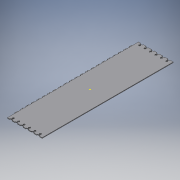
# Autodesk Inventor part: 3DPrinterBracket_bottom
Saved by Autodesk Inventor 2016 (Build 200138000, 138)
## iProperties
Created: 2017-10-03
Part Number: 3DPrinterBracket_bottom
Material: Generic
Document SubType Name: Modeling
Designer: jcj2131
Density: 1 g/cm^3
Appearance: Default
Author: jcj2131
Autodesk Inventor part; units mm, degrees
ref_plane "YZ Plane" through (0, 0, 0) normal (1, 0, 0) x (0, 1, 0)
ref_plane "XZ Plane" through (0, 0, 0) normal (0, 1, 0) x (-1, 0, 0)
ref_plane "XY Plane" through (0, 0, 0) normal (0, 0, 1) x (1, 0, 0)
sketch "Sketch1" plane through (0, 0, 0) normal (0, 1, 0) x (-1, 0, 0)
  line L0 (82.55, 306.3875) -> (-82.55, 306.3875)
  line L1 (-82.55, 306.3875) -> (-82.55, -306.3875)
  line L2 (-82.55, -306.3875) -> (82.55, -306.3875)
  line L3 (82.55, -306.3875) -> (82.55, 306.3875)
  point P0 (0, 0)
  point P1 (0, 306.3875)
  point P2 (82.55, 0)
  dimension "d0" = 612.775
  dimension "d1" = 165.1
  constraints: 8 end point, 2 midpoint, 2 parallel, 1 horizontal, 1 horizontal alignment, 1 perpendicular, 1 vertical alignment
  measures "d0" distance of L2.end L0.start
  measures "d1" distance of L0.start L0.end
extrude "Extrusion1" add sketch "Sketch1" along normal blind 3.175
sketch "Sketch2" plane through (0, 3.175, 0) normal (0, 1, 0) x (1, 0, 0)
  line L0 (-82.55, -306.3875) -> (82.55, -306.3875) projected
  line L1 (-69.85, -306.3875) -> (-57.15, -306.3875)
  line L2 (-57.15, -306.3875) -> (-57.15, -303.2125)
  line L3 (-57.15, -303.2125) -> (-69.85, -303.2125)
  line L4 (-69.85, -303.2125) -> (-69.85, -306.3875)
  line L5 (-82.55, 306.3875) -> (-82.55, -306.3875) projected
  point P0 (0, 0)
  dimension "d4" = 12.7
  dimension "d5" = 12.7
  dimension "d6" = 3.175
  constraints: 8 end point, 2 parallel, 1 horizontal, 1 perpendicular, 1 point on line
  measures "d4" distance between parallel lines of L5 L4
  measures "d5" distance of L2.end L3.end
  measures "d6" distance of L1.end L2.end
extrude "Extrusion2" cut sketch "Sketch2" against normal through all
sketch "Sketch3" plane through (0, 3.175, 0) normal (0, 1, 0) x (1, 0, 0)
  line L0 (-57.15, -303.2125) -> (-69.85, -303.2125) projected
  line L1 (-65.278, -303.2125) -> (-61.722, -303.2125)
  line L2 (-61.722, -303.2125) -> (-61.722, -297.2125)
  line L3 (-61.722, -297.2125) -> (-65.278, -297.2125)
  line L4 (-65.278, -297.2125) -> (-65.278, -303.2125)
  line L5 (-69.85, -306.3875) -> (-69.85, -303.2125) projected
  point P0 (0, 0)
  dimension "d9" = 3.556
  dimension "d10" = 6
  dimension "d11" = 4.572
  constraints: 8 end point, 2 parallel, 1 horizontal, 1 perpendicular, 1 point on line
  measures "d9" distance of L2.end L3.end
  measures "d10" distance of L3.end L1.start
  measures "d11" distance between parallel lines of L5 L4
extrude "Extrusion3" cut sketch "Sketch3" against normal through all
sketch "Sketch4" plane through (0, 3.175, 0) normal (0, 1, 0) x (1, 0, 0)
  line L0 (-59.5315, -297.2125) -> (-67.469, -297.2125)
  line L1 (-67.469, -297.2125) -> (-67.469, -294.4345)
  line L2 (-67.469, -294.4345) -> (-59.5315, -294.4345)
  line L3 (-59.5315, -294.4345) -> (-59.5315, -297.2125)
  line L4 (-65.278, -297.2125) -> (-61.722, -297.2125) projected
  line L5 (-69.85, -306.3875) -> (-69.85, -303.2125) projected
  point P0 (0, 0)
  dimension "d14" = 7.9375
  dimension "d15" = 2.778
  dimension "d16" = 0
  dimension "d17" = 2.381
  constraints: 8 end point, 2 parallel, 1 horizontal, 1 perpendicular
  measures "d14" distance of L1.end L2.end
  measures "d15" distance of L0.end L1.end
  measures "d16" distance between parallel lines of L4 L0
  measures "d17" distance between parallel lines of L5 L1
extrude "Extrusion4" cut sketch "Sketch4" against normal through all
sketch "Sketch5" plane through (0, 3.175, 0) normal (0, 1, 0) x (1, 0, 0)
  line L0 (-59.5315, -294.4345) -> (-67.469, -294.4345) projected
  line L1 (-65.278, -294.4345) -> (-61.722, -294.4345)
  line L2 (-61.722, -294.4345) -> (-61.722, -291.1475)
  line L3 (-61.722, -291.1475) -> (-65.278, -291.1475)
  line L4 (-65.278, -291.1475) -> (-65.278, -294.4345)
  line L5 (-69.85, -306.3875) -> (-69.85, -303.2125) projected
  line L6 (-57.15, -306.3875) -> (82.55, -306.3875) projected
  point P0 (0, 0)
  dimension "d20" = 3.556
  dimension "d21" = 4.572
  dimension "d22" = 15.24
  constraints: 8 end point, 2 parallel, 1 horizontal, 1 perpendicular, 1 point on line
  measures "d20" distance of L2.end L3.end
  measures "d21" distance between parallel lines of L5 L4
  measures "d22" distance between parallel lines of L6 L3
extrude "Extrusion5" cut sketch "Sketch5" against normal through all
pattern_linear "Rectangular Pattern1" count 6 spacing 25.4 along (1, 0, 0) of "Extrusion2", "Extrusion3", "Extrusion4", "Extrusion5"
sketch "Sketch6" plane through (0, 3.175, 0) normal (0, 1, 0) x (1, 0, 0)
  point P0 (0, 0)
mirror "Mirror1" about plane through (0, 0, 0) normal (0, 0, 1) of "Extrusion5", "Extrusion2", "Extrusion3", "Extrusion4", "Rectangular Pattern1"
sketch "Sketch18" plane through (0, 3.175, 0) normal (0, 1, 0) x (1, 0, 0)
  line L0 (-46.25, 241.3875) -> (-6.25, 241.3875)
  line L1 (-6.25, 241.3875) -> (-6.25, 281.3875)
  line L2 (-6.25, 281.3875) -> (-46.25, 281.3875)
  line L3 (-46.25, 281.3875) -> (-46.25, 241.3875)
  line L4 (82.55, -306.3875) -> (82.55, 306.3875) projected
  line L5 (-19.05, 306.3875) -> (-31.75, 306.3875) projected
  point P0 (0, 0)
  dimension "d120" = 40
  dimension "d121" = 40
  dimension "d122" = 128.8
  dimension "d123" = 25
  constraints: 8 end point, 2 parallel, 1 horizontal, 1 perpendicular
  measures "d120" distance of L2.end L0.start
  measures "d121" distance of L1.end L2.end
  measures "d122" distance between parallel lines of L4 L3
  measures "d123" distance between parallel lines of L5 L2
extrude "Extrusion13" [suppressed]
sketch "Sketch19" plane through (0, 3.175, 0) normal (0, 1, 0) x (1, 0, 0)
  circle A0 centre (-60.6, 251.3875) radius 2.75
  line L0 (-6.25, 241.3875) -> (-46.25, 241.3875) projected
  circle A1 centre (-60.6, 271.3875) radius 2.75
  line L1 (-46.25, 281.3875) -> (-46.25, 241.3875) projected
  point P0 (0, 0)
  dimension "d126" = 5.5
  dimension "d127" = 10
  dimension "d128" = 5.5
  dimension "d129" = 20
  dimension "d130" = 14.35
  dimension "d131" = 14.35
  constraints: 2 centre point
  measures "d126" diameter of A0
  measures "d127" distance from line of L0 A0.centre
  measures "d128" diameter of A1
  measures "d129" distance of A0.centre A1.centre
  measures "d130" distance from line of L1 A0.centre
  measures "d131" distance from line of L1 A1.centre
extrude "Extrusion14" [suppressed]
sketch "Sketch20" plane through (0, 3.175, 0) normal (0, 1, 0) x (1, 0, 0)
  line L0 (-82.55, -306.3875) -> (-69.85, -306.3875) projected
  line L1 (-82.55, -306.3875) -> (-79.375, -306.3875)
  line L2 (-79.375, -306.3875) -> (-79.375, -268.2875)
  line L3 (-79.375, -268.2875) -> (-82.55, -268.2875)
  line L4 (-82.55, -268.2875) -> (-82.55, -306.3875)
  line L5 (-82.55, 306.3875) -> (-82.55, -306.3875) projected
  line L6 (-82.55, -263.7155) -> (-79.375, -263.7155)
  line L7 (-79.375, -263.7155) -> (-79.375, -260.1595)
  line L8 (-79.375, -260.1595) -> (-82.55, -260.1595)
  line L9 (-82.55, -260.1595) -> (-82.55, -263.7155)
  point P0 (0, 0)
  dimension "d134" = 3.175
  dimension "d135" = 38.1
  dimension "d136" = 4.572
  dimension "d137" = 3.556
  constraints: 16 end point, 4 parallel, 2 horizontal, 2 perpendicular, 1 collinear, 1 point on line
  measures "d134" distance of L2.end L3.end
  measures "d135" distance of L1.end L2.end
  measures "d136" distance between parallel lines of L3 L6
  measures "d137" distance of L6.end L7.end
extrude "Extrusion15" cut sketch "Sketch20" against normal through all
sketch "Sketch21" plane through (0, 3.175, 0) normal (0, 1, 0) x (1, 0, 0)
  line L0 (-82.55, 306.3875) -> (-82.55, -260.1595) projected
  line L1 (-82.55, -255.5875) -> (-79.375, -255.5875)
  line L2 (-79.375, -255.5875) -> (-79.375, -242.8875)
  line L3 (-79.375, -242.8875) -> (-82.55, -242.8875)
  line L4 (-82.55, -242.8875) -> (-82.55, -255.5875)
  line L5 (-82.55, -260.1595) -> (-79.375, -260.1595) projected
  line L6 (-82.55, -238.2905) -> (-79.375, -238.2905)
  line L7 (-79.375, -238.2905) -> (-79.375, -234.7345)
  line L8 (-79.375, -234.7345) -> (-82.55, -234.7345)
  line L9 (-82.55, -234.7345) -> (-82.55, -238.2905)
  point P0 (0, 0)
  dimension "d140" = 3.175
  dimension "d141" = 4.572
  dimension "d142" = 12.7
  dimension "d143" = 4.597
  dimension "d144" = 3.556
  constraints: 16 end point, 4 parallel, 2 horizontal, 2 perpendicular, 2 point on line
  measures "d140" distance of L2.end L3.end
  measures "d141" distance between parallel lines of L5 L1
  measures "d142" distance of L1.end L2.end
  measures "d143" distance between parallel lines of L3 L6
  measures "d144" distance of L6.end L7.end
extrude "Extrusion16" cut sketch "Sketch21" against normal through all
pattern_linear "Rectangular Pattern3" count 21 spacing 25.4 along (0, 0, -1) of "Extrusion16"
sketch "Sketch22" plane through (0, 3.175, 0) normal (0, 1, 0) x (1, 0, 0)
  line L0 (-82.55, 306.3875) -> (-79.375, 306.3875)
  line L1 (-79.375, 306.3875) -> (-79.375, 277.7875)
  line L2 (-79.375, 277.7875) -> (-82.55, 277.7875)
  line L3 (-82.55, 277.7875) -> (-82.55, 306.3875)
  line L4 (-82.55, 273.2655) -> (-79.375, 273.2655) projected
  point P0 (0, 0)
  dimension "d150" = 3.175
  dimension "d154" = 28.6
  constraints: 8 end point, 2 parallel, 1 horizontal, 1 perpendicular
  measures "d150" distance of L1.end L2.end
  measures "d154" distance of L0.end L1.end
extrude "Extrusion17" cut sketch "Sketch22" against normal through all
body "Solid1"
